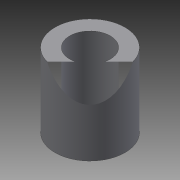
# Autodesk Inventor part: cuscinetto_X
Saved by Autodesk Inventor 2014 SP1 (Build 180222100, 222)
## iProperties
Created: 2015-04-08
Part Number: cuscinetto_X
Material: Generic
Document SubType Name: Modeling
Designer: Giorgio Nuzzo
Density: 1 g/cm^3
Appearance: Default
d0: 20,000 mm
d1: 0,00 deg
d2: 4,000 mm
Author: Giorgio Nuzzo
Autodesk Inventor part; units mm, degrees
ref_plane "YZ Plane" through (0, 0, 0) normal (1, 0, 0) x (0, 1, 0)
ref_plane "XZ Plane" through (0, 0, 0) normal (0, 1, 0) x (-1, 0, 0)
ref_plane "XY Plane" through (0, 0, 0) normal (0, 0, 1) x (1, 0, 0)
sketch "Sketch1" plane through (0, 0, 0) normal (0, 0, 1) x (1, 0, 0)
  circle A0 centre (0, 2.195) radius 7.5 projected
  circle A1 centre (0, 2.195) radius 3.5
  point P0 (0, 0)
  dimension "d2" = 4
  constraints: 1 centre point
  measures "d2" radial gap between concentric circles of A0 A1
extrude "Extrusion1" add sketch "Sketch1" along normal mid plane 20
body "Solid1"
